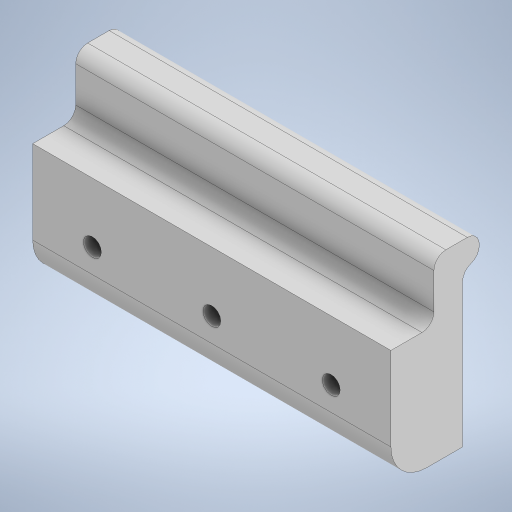
# Autodesk Inventor part: paliczek_v2
Saved by Autodesk Inventor 2024.2 (Build 282272000, 272)
## iProperties
Created: 2024-01-13
Part Number: paliczek_v2
Material: PLA
Document SubType Name: Modeling
Designer: Konrad
Density: 1 g/cm^3
Appearance: Domyślna
Author: Konrad
Autodesk Inventor part; units mm, degrees
ref_plane "YZ Plane" through (0, 0, 0) normal (1, 0, 0) x (0, 1, 0)
ref_plane "XZ Plane" through (0, 0, 0) normal (0, 1, 0) x (-1, 0, 0)
ref_plane "XY Plane" through (0, 0, 0) normal (0, 0, 1) x (1, 0, 0)
sketch "Szkic1" plane through (0, 0, 0) normal (1, 0, 0) x (0, 1, 0)
  line L0 (0, 0) -> (10, 0)
  line L1 (10, 0) -> (10, -3.6)
  line L2 (10, -3.6) -> (15, -3.6)
  line L3 (15, -3.6) -> (15, -7.4)
  line L4 (15, -7.4) -> (13, -7.4)
  line L5 (13, -7.4) -> (13, -6)
  line L6 (13, -6) -> (0, -6)
  line L7 (0, -6) -> (0, 0)
  dimension "d1" = 2.4
  dimension "d2" = 3.8
  dimension "d3" = 2
  dimension "d4" = 3.6
  dimension "d5" = 5
  dimension "d6" = 15
  constraints: 16 end point, 7 perpendicular, 1 horizontal
  measures "d1" distance between parallel lines of L2 L6
  measures "d2" distance of L2.end L3.end
  measures "d3" distance of L3.end L4.end
  measures "d4" distance of L0.end L1.end
  measures "d5" distance of L1.end L2.end
  measures "d6" distance between parallel lines of L7 L3
extrude "Wyciągnięcie proste1" add sketch "Szkic1" along normal blind 30
fillet "Zaokrąglenie1" radius 3 1 edges at (15, 0, 0)
fillet "Zaokrąglenie2" radius 1 5 edges at (15, 15, -3.6) (15, 10, -3.6) (15, 15, -7.4) (15, 13, -7.4) (15, 13, -6)
sketch "Szkic4" plane through (0, 10, 0) normal (0, 0, 1) x (1, 0, 0)
  line L0 (30, -7) -> (0, -7) projected
  line L1 (30, 0) -> (30, -7) projected
  line L2 (0, 0) -> (30, 0) construction
  line L3 (0, 0) -> (0, -7) projected
  circle A0 centre (25, -5) radius 0.75
  circle A1 centre (15, -5) radius 0.75
  circle A2 centre (5, -5) radius 0.75
  dimension "d27" = 1.5
  dimension "d28" = 2
  dimension "d32" = 10
  dimension "d38" = 30
  dimension "d39" = 15
  constraints: 3 centre point, 1 horizontal, 4 other
  measures "d27" diameter of A0
  measures "d28" distance from line of L0 A0.centre
  measures "d32" distance of A0.centre A1.centre
  measures "d38" distance of L0.start L0.end
  measures "d39" distance from line of A1.centre L1
extrude "Wyciągnięcie proste5" cut sketch "Szkic4" against normal through all
equation "\"d39\" = 0.5 * d38"
